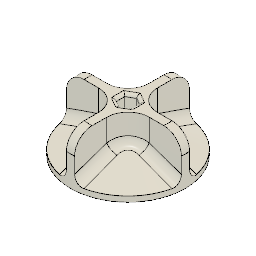
Carousel-3 (Autodesk Fusion 360 design; units mm, degrees)
Autodesk Fusion 360 part; units mm, degrees
sketch "Sketch1" plane through (0, 0, 0) normal (0, 1, 0) x (1, 0, 0)
  circle A0 centre (0, 0) radius 49
  dimension "d1" = 98
  constraint coincident A0.centre origin
  measures "d1" diameter of A0
extrude "Extrude1" add sketch "Sketch1" along normal blind 5
chamfer "Chamfer1" distance 0.5 angle 45 1 edges at (-45.684, 0, 17.7192)
sketch "Sketch2" plane through (0, 5, 0) normal (0, 1, 0) x (-1, 0, 0)
  circle A0 centre (0, 0) radius 49
  circle A1 centre (0, 0) radius 4.1
  line L0 (-52.9671, -3.5) -> (52.9671, -3.5)
  line L1 (52.9671, -3.5) -> (52.9671, 3.5)
  line L2 (52.9671, 3.5) -> (-52.9671, 3.5)
  line L3 (-52.9671, 3.5) -> (-52.9671, -3.5)
  line L4 (-52.9671, -3.5) -> (52.9671, 3.5) construction
  line L5 (52.9671, -3.5) -> (-52.9671, 3.5) construction
  line L6 (-3.5, -53.3296) -> (3.5, -53.3296)
  line L7 (3.5, -53.3296) -> (3.5, 53.3296)
  line L8 (3.5, 53.3296) -> (-3.5, 53.3296)
  line L9 (-3.5, 53.3296) -> (-3.5, -53.3296)
  line L10 (-3.5, -53.3296) -> (3.5, 53.3296) construction
  line L11 (3.5, -53.3296) -> (-3.5, 53.3296) construction
  circle A2 centre (21.5, -21.5) radius 18
  circle A3 centre (-21.5, -21.5) radius 18
  circle A4 centre (-21.5, 21.5) radius 18
  circle A5 centre (21.5, 21.5) radius 18
  dimension "d5" = 8.2
  dimension "d6" = 7
  dimension "d7" = 7
  dimension "d8" = 18
  dimension "d9" = 18
  dimension "d10" = 18
  dimension "d11" = 18
  constraint coincident A0.centre A1.centre
  constraint perpendicular L0 L1
  constraint parallel L0 L2
  constraint parallel L1 L3
  constraint horizontal L0
  constraint coincident L4 A0.centre
  constraint coincident L5 A0.centre
  constraint perpendicular L6 L7
  constraint parallel L6 L8
  constraint parallel L7 L9
  constraint horizontal L6
  constraint coincident L10 A0.centre
  constraint coincident L11 A0.centre
  constraint tangent L0 A2
  constraint tangent L7 A2
  constraint tangent L9 A3
  constraint tangent L0 A3
  constraint tangent L2 A4
  constraint tangent L9 A4
  constraint tangent L2 A5
  constraint tangent L7 A5
  measures "d5" diameter of A1
  measures "d6" distance of L0.end L1.end
  measures "d7" distance of L7.end L8.end
  measures "d8" radius of A2
  measures "d9" radius of A3
  measures "d10" radius of A4
  measures "d11" radius of A5
extrude "Extrude2" add sketch "Sketch2" along normal blind 36 contours A0 A1 L0 L2 L7 | A0 A1 L2 L7 L9 | L2 L7 A5 | A0 A1 L0 L7 L9 | L0 L7 A2 | A1 L2 L7 | A1 L0 L7 | A0 A1 L0 L2 L9 | L2 L9 A4 | L0 L9 A3 | A1 L2 L9 | A1 L0 L9
sketch "Sketch3" plane through (0, 41, 0) normal (0, 1, 0) x (-1, 0, 0)
  circle A0 centre (0, 0) radius 4.1
  arc A1 (48.8748, -3.5) -> (48.8748, 3.5) centre (0, 0) ccw
  line L0 (48.8748, 3.5) -> (21.5, 3.5)
  arc A2 (3.5, 21.5) -> (21.5, 3.5) centre (21.5, 21.5) ccw
  line L1 (3.5, 21.5) -> (3.5, 48.8748)
  arc A3 (3.5, 48.8748) -> (-3.5, 48.8748) centre (0, 0) ccw
  line L2 (-3.5, 48.8748) -> (-3.5, 21.5)
  arc A4 (-21.5, 3.5) -> (-3.5, 21.5) centre (-21.5, 21.5) ccw
  line L3 (-21.5, 3.5) -> (-48.8748, 3.5)
  arc A5 (-48.8748, 3.5) -> (-48.8748, -3.5) centre (0, 0) ccw
  line L4 (-48.8748, -3.5) -> (-21.5, -3.5)
  arc A6 (-3.5, -21.5) -> (-21.5, -3.5) centre (-21.5, -21.5) ccw
  line L5 (-3.5, -21.5) -> (-3.5, -48.8748)
  arc A7 (-3.5, -48.8748) -> (3.5, -48.8748) centre (0, 0) ccw
  line L6 (3.5, -48.8748) -> (3.5, -21.5)
  arc A8 (21.5, -3.5) -> (3.5, -21.5) centre (21.5, -21.5) ccw
  line L7 (21.5, -3.5) -> (48.8748, -3.5)
  line L8 (0, -7.5) -> (6.4952, -3.75)
  line L9 (6.4952, -3.75) -> (6.4952, 3.75)
  line L10 (6.4952, 3.75) -> (0, 7.5)
  line L11 (0, 7.5) -> (-6.4952, 3.75)
  line L12 (-6.4952, 3.75) -> (-6.4952, -3.75)
  line L13 (-6.4952, -3.75) -> (0, -7.5)
  dimension "d14" = 7.5
  constraint coincident A0.centre A1.centre
  measures "d14" distance of L8.start A0.centre
extrude "Extrude3" cut sketch "Sketch3" against normal blind 15 contours L8 L9 L10 L11 L12 L13
extrude "Extrude4" cut 1 faces at (1.7873, 5, -1.1088) along direction (0, -1, 0) blind 5
ref_plane "WorkPlane1" through (35.1874, 23, 0) normal (0, 0, 1) x (1, 0, 0)
sketch "Sketch4" plane through (35.1874, 23, 0) normal (0, 0, 1) x (1, 0, 0)
  line L0 (-31.0874, -23) -> (-39.2874, -23)
  line L1 (-31.0874, 3) -> (-39.2874, 3)
  line L2 (-28.6922, 18) -> (-35.1874, 18)
  line L3 (-35.1874, 18) -> (-35.1874, 3)
  line L4 (-35.1874, 3) -> (-28.6922, 3)
  line L5 (-28.6922, 3) -> (-28.6922, 18)
  line L6 (-35.1874, 18) -> (-41.6826, 18)
  line L7 (-41.6826, 18) -> (-41.6826, 3)
  line L8 (-41.6826, 3) -> (-35.1874, 3)
  line L9 (-35.1874, 3) -> (-35.1874, 18)
  line L10 (13.6874, -18) -> (-13.6874, -18)
  line L11 (-13.6874, -18) -> (-13.6874, 18)
  line L12 (-13.6874, 18) -> (13.6874, 18)
  line L13 (13.6874, 18) -> (13.6874, -18)
  line L14 (-13.6874, -18) -> (-31.6874, -18)
  line L15 (-31.6874, -18) -> (-31.6874, 18)
  line L16 (-31.6874, 18) -> (-13.6874, 18)
  line L17 (-13.6874, 18) -> (-13.6874, -18)
  line L18 (-31.0874, -23) -> (-39.2874, -23)
  line L19 (13.3126, -23) -> (-83.6874, -23)
  line L20 (-28.6922, 18) -> (-35.1874, 18)
  line L21 (-35.1874, 18) -> (-35.1874, -23)
  line L22 (-35.1874, -23) -> (-28.6922, -23)
  line L23 (-28.6922, -23) -> (-28.6922, 18)
  line L24 (13.3126, -23) -> (13.6874, -18)
  line L25 (13.3126, -23) -> (-31.0874, -23)
  line L26 (13.6874, -18) -> (-28.6922, -2.5)
  constraint horizontal L20
  constraint vertical L21
  constraint horizontal L22
  constraint vertical L23
  constraint midpoint L18 L21.end
  constraint coincident L2.start L5.end
  constraint coincident L10.start L13.end
  constraint coincident L19.start L24.start
  constraint coincident L0.start L18.start
  constraint midpoint L23 L26.end
revolve "Revolve1" add sketch "Sketch4" angle 360 about axis through (0, 41, 0) along (0, -1, 0) contours L11 L14 L17 L23 L26 | L10 L11 L17 L26
fillet "Fillet4" radius 7.5 12 edges at (31.6024, 11.2466, 3.5) (8.7721, 18.3383, 8.7721) (3.5, 11.2466, 31.6024) (-3.5, 11.2466, 31.6024) (-8.7721, 18.3383, 8.7721) (-31.6024, 11.2466, 3.5) (-31.6024, 11.2466, -3.5) (-8.7721, 18.3383, -8.7721) (-3.5, 11.2466, -31.6024) (3.5, 11.2466, -31.6024) (8.7721, 18.3383, -8.7721) (31.6024, 11.2466, -3.5)
fillet "Fillet1" radius 15 4 edges at (-49, 41, 0) (0, 41, -49) (49, 41, 0) (0, 41, 49)
fillet "Fillet3" radius 2.5 6 edges at (-3.2476, 41, -5.625) (-6.4952, 41, 0) (-3.2476, 41, 5.625) (3.2476, 41, 5.625) (6.4952, 41, 0) (3.2476, 41, -5.625)
sketch "Sketch6" plane through (35.1874, 23, 0) normal (0, 0, 1) x (1, 0, 0)
  line L0 (13.3126, -23) -> (-83.6874, -23)
  line L1 (-84.1874, -22.5) -> (13.8126, -22.5)
  line L2 (-31.6874, 3) -> (-38.6874, 3)
  line L3 (-38.6874, 3) -> (-38.6874, -10.4613)
  spline S0 degree 3 poles (-44.8619, -18) (-44.259, -17.9284) (-43.6667, -17.773) (-42.3101, -17.2012) (-41.5944, -16.718) (-40.3172, -15.4635) (-39.7869, -14.6881) (-39.1672, -13.3124) (-38.9883, -12.761) (-38.7477, -11.626) (-38.6874, -11.0441) (-38.6874, -10.4613) knots 0.079821 0.079821 0.079821 0.079821 0.267032 0.267032 0.526783 0.526783 0.806302 0.806302 0.979417 0.979417 1.154063 1.154063 1.154063 1.154063
  line L4 (-44.8619, -18) -> (-83.2229, -18)
  spline S1 degree 3 poles (-84.0623, -10.4613) (-84.0623, -11.5517) (-84.0485, -12.6359) (-83.9807, -14.5546) (-83.9302, -15.3904) (-83.7718, -16.7185) (-83.6707, -17.2202) (-83.4442, -17.7837) (-83.3401, -17.9309) (-83.2229, -18) knots 0 0 0 0 0.327127 0.327127 0.625191 0.625191 0.896226 0.896226 1.077333 1.077333 1.077333 1.077333
  line L5 (-84.0623, -10.4613) -> (-84.0623, 3)
  line L6 (-84.0623, 3) -> (-84.1874, 3)
  line L7 (-84.0623, 3) -> (-84.0623, -10.4613)
  spline S2 degree 3 poles (-83.2229, -18) (-83.3443, -17.9284) (-83.4516, -17.773) (-83.6736, -17.2012) (-83.7707, -16.718) (-83.9227, -15.4635) (-83.9726, -14.6881) (-84.0261, -13.3124) (-84.0399, -12.761) (-84.0581, -11.626) (-84.0623, -11.0441) (-84.0623, -10.4613) knots 0.079821 0.079821 0.079821 0.079821 0.267032 0.267032 0.526783 0.526783 0.806302 0.806302 0.979417 0.979417 1.154063 1.154063 1.154063 1.154063
  line L8 (-44.8619, -18) -> (-83.2229, -18)
  spline S3 degree 3 poles (-38.6874, -10.4613) (-38.6874, -11.5517) (-38.8985, -12.6359) (-39.7002, -14.5546) (-40.2508, -15.3904) (-41.5879, -16.7185) (-42.3338, -17.2202) (-43.7078, -17.7837) (-44.28, -17.9309) (-44.8619, -18) knots 0 0 0 0 0.327127 0.327127 0.625191 0.625191 0.896226 0.896226 1.077333 1.077333 1.077333 1.077333
  line L9 (-38.6874, -10.4613) -> (-38.6874, 3)
  line L10 (-31.6874, 3) -> (-38.6874, 3)
  line L11 (-31.6874, 3) -> (-31.6874, -10.4613)
  spline S4 degree 3 poles (-25.5129, -18) (-26.1159, -17.9284) (-26.7082, -17.773) (-28.0647, -17.2012) (-28.7805, -16.718) (-30.0576, -15.4635) (-30.588, -14.6881) (-31.2076, -13.3124) (-31.3865, -12.761) (-31.6271, -11.626) (-31.6874, -11.0441) (-31.6874, -10.4613) knots 0.079821 0.079821 0.079821 0.079821 0.267032 0.267032 0.526783 0.526783 0.806302 0.806302 0.979417 0.979417 1.154063 1.154063 1.154063 1.154063
  line L12 (12.848, -18) -> (-25.5129, -18)
  spline S5 degree 3 poles (13.6874, -10.4613) (13.6874, -11.5517) (13.6737, -12.6359) (13.6058, -14.5546) (13.5554, -15.3904) (13.397, -16.7185) (13.2958, -17.2202) (13.0693, -17.7837) (12.9652, -17.9309) (12.848, -18) knots 0 0 0 0 0.327127 0.327127 0.625191 0.625191 0.896226 0.896226 1.077333 1.077333 1.077333 1.077333
  line L13 (13.6874, -10.4613) -> (13.6874, 3)
  line L14 (13.8126, 3) -> (13.6874, 3)
  line L15 (13.6874, 3) -> (13.6874, -10.4613)
  spline S6 degree 3 poles (12.848, -18) (12.9695, -17.9284) (13.0768, -17.773) (13.2987, -17.2012) (13.3959, -16.718) (13.5479, -15.4635) (13.5977, -14.6881) (13.6513, -13.3124) (13.6651, -12.761) (13.6832, -11.626) (13.6874, -11.0441) (13.6874, -10.4613) knots 0.079821 0.079821 0.079821 0.079821 0.267032 0.267032 0.526783 0.526783 0.806302 0.806302 0.979417 0.979417 1.154063 1.154063 1.154063 1.154063
  line L16 (12.848, -18) -> (-25.5129, -18)
  spline S7 degree 3 poles (-31.6874, -10.4613) (-31.6874, -11.5517) (-31.4764, -12.6359) (-30.6746, -14.5546) (-30.1241, -15.3904) (-28.787, -16.7185) (-28.041, -17.2202) (-26.667, -17.7837) (-26.0948, -17.9309) (-25.5129, -18) knots 0 0 0 0 0.327127 0.327127 0.625191 0.625191 0.896226 0.896226 1.077333 1.077333 1.077333 1.077333
  line L17 (-31.6874, -10.4613) -> (-31.6874, 3)
  line L18 (-84.1874, -22.5) -> (13.8126, -22.5)
  line L19 (13.3126, -23) -> (9.3126, -23)
  line L20 (9.3126, -23) -> (4.5126, -23)
  line L21 (9.3126, -23) -> (4.5126, -23)
  line L22 (4.5126, -23) -> (4.5126, -19.5)
  line L23 (4.5126, -19.5) -> (9.3126, -19.5)
  line L24 (9.3126, -19.5) -> (9.3126, -23)
  circle A0 centre (6.9126, -21.75) radius 2.25
  line L25 (6.9126, -21.75) -> (6.9126, -18.5)
  line L26 (6.9126, -18.5) -> (5.289, -20.1923)
  line L27 (6.9126, -18.5) -> (8.5362, -20.1923)
  line L28 (8.5362, -20.1923) -> (9.3126, -21.0016)
  line L29 (5.289, -20.1923) -> (4.5126, -21.0016)
  point P0 (9.3126, -23)
  dimension "d31" = 4
  dimension "d32" = 4.8
  dimension "d33" = 3.5
  dimension "d34" = 4.5
  dimension "d35" = 3.25
  constraint coincident L0.start L19.start
  constraint parallel L0 L19
  constraint parallel L0 L20
  constraint coincident P0 L19.end
  constraint horizontal L21
  constraint vertical L22
  constraint horizontal L23
  constraint vertical L24
  constraint coincident A0.centre L25.start
  constraint vertical L25
  constraint coincident A0 L26.end
  constraint tangent A0 L26
  constraint coincident A0 L27.end
  constraint tangent A0 L27
  constraint coincident L24 L28.end
  constraint tangent A0 L28
  constraint coincident L22 L29.end
  constraint tangent A0 L29
  measures "d31" distance of L0.start P0
  measures "d32" distance of P0 L20.end
  measures "d33" distance of P0 L23.end
  measures "d34" diameter of A0
  measures "d35" distance of A0.centre L25.end
revolve "Revolve3" cut sketch "Sketch6" angle 360 about axis through (0, 1.75, 0) along (0, 1, 0) contours L0 L1 L18 L20 L21 L24 A0 | L0 L20 L21 A0 | L0 L1 L18 L20 L21 A0 | L1 L18 L24 A0 L28 | L0 L1 L18 L20 L21 L22 A0 | L1 L18 A0 | L1 L18 L22 A0 L29 | L23 A0 L27 | L23 A0 L26 | L23 L25 L27 | L23 L25 L26
chamfer "Chamfer3" distance 0.5 angle 45 2 edges at (-37.0134, 0, -14.3561) (-41.4886, 0, 16.0919)
chamfer "Chamfer4" distance 0.5 angle 45 1 edges at (3.8225, 0, -1.4826)
equation "d14 = ( 15 / 2 ) * 1 mm"
